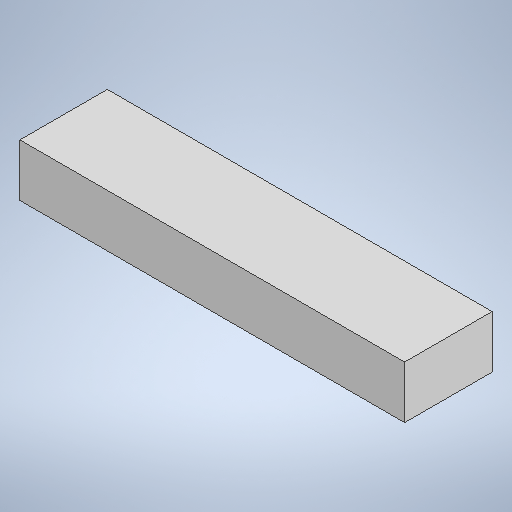
# Autodesk Inventor part: block
Saved by Autodesk Inventor 2025.1 (Build 291241020, 241B)
## iProperties
Created: 2025-03-17
Part Number: block
Material: Generic
Document SubType Name: Modeling
Designer: omiye
Density: 1 g/cm^3
Appearance: Default
Author: omiye
Autodesk Inventor part; units mm, degrees
ref_plane "YZ Plane" through (0, 0, 0) normal (1, 0, 0) x (0, 1, 0)
ref_plane "XZ Plane" through (0, 0, 0) normal (0, 1, 0) x (-1, 0, 0)
ref_plane "XY Plane" through (0, 0, 0) normal (0, 0, 1) x (1, 0, 0)
sketch "Sketch1" plane through (0, 0, 0) normal (0, 1, 0) x (-1, 0, 0)
  line L0 (-16.5, -3.75) -> (-16.5, 3.75)
  line L1 (-16.5, 3.75) -> (16.5, 3.75)
  line L2 (16.5, 3.75) -> (16.5, -3.75)
  line L3 (16.5, -3.75) -> (-16.5, -3.75)
  line L4 (-16.5, -3.75) -> (16.5, 3.75) construction
  line L5 (-16.5, 3.75) -> (16.5, -3.75) construction
  point P0 (0, 0)
  dimension "d0" = 7.5
  dimension "d1" = 33
  constraints: 12 end point, 2 midpoint, 2 parallel, 1 perpendicular, 1 vertical
  measures "d0" distance of L0.start L0.end
  measures "d1" distance of L0.end L1.end
extrude "Extrusion1" add sketch "Sketch1" along normal blind 4.5
body "Solid1"
